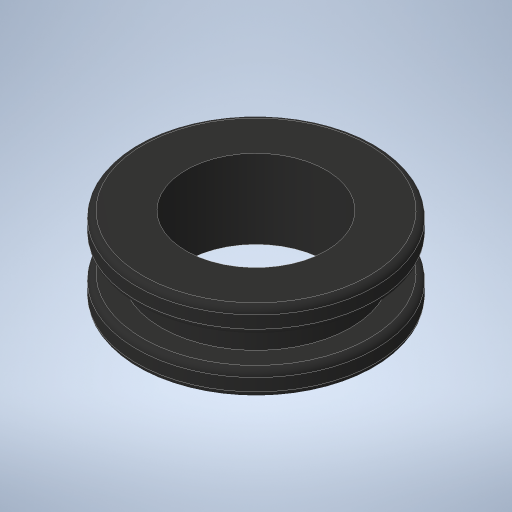
# Autodesk Inventor part: .5 tpu grommet
Saved by Autodesk Inventor 2023.4 (Build 274418000, 418)
## iProperties
Created: 2025-03-24
Part Number: .5 tpu grommet
Material: Rubber, Black
Document SubType Name: Modeling
Designer: jmcintyr
Density: 0.93 g/cm^3
Appearance: Rubber - Black
Author: jmcintyr
Autodesk Inventor part; units mm, degrees
ref_plane "YZ Plane" through (0, 0, 0) normal (1, 0, 0) x (0, 1, 0)
ref_plane "XZ Plane" through (0, 0, 0) normal (0, 1, 0) x (-1, 0, 0)
ref_plane "XY Plane" through (0, 0, 0) normal (0, 0, 1) x (1, 0, 0)
sketch "Sketch1" plane through (0, 0, 0) normal (0, 0, 1) x (1, 0, 0)
  line L0 (4.5085, 2.54) -> (4.5085, -2.54)
  line L1 (4.5085, -2.54) -> (7.6835, -2.54)
  line L2 (7.6835, -2.54) -> (7.6835, -0.9525)
  line L3 (7.6835, -0.9525) -> (6.096, -0.9525)
  line L4 (6.096, -0.9525) -> (6.096, 0.9525)
  line L5 (6.096, 0.9525) -> (7.6835, 0.9525)
  line L6 (7.6835, 0.9525) -> (7.6835, 2.54)
  line L7 (7.6835, 2.54) -> (4.5085, 2.54)
  line L8 (0, 0) -> (0, 2.54) construction
  point P0 (4.5085, 0)
  point P1 (6.096, 0)
  dimension "d0" = 6.096
  dimension "d1" = 1.905
  dimension "d2" = 5.08
  dimension "d3" = 1.5875
  dimension "d4" = 1.5875
  dimension "d5" = 1.5875
  constraints: 18 end point, 7 perpendicular, 3 horizontal alignment, 2 midpoint, 2 vertical, 1 vertical alignment
  measures "d0" distance from line of L8.start L4
  measures "d1" distance of L3.end L4.end
  measures "d2" distance of L0.start L0.end
  measures "d3" distance of L5.end L6.end
  measures "d4" distance between parallel lines of L4 L0
  measures "d5" distance of L2.end L3.end
revolve "Revolution1" add sketch "Sketch1" angle 360 about axis through (0, 0, 0) along (0, 1, 0)
fillet "Fillet1" radius 0.3969 4 edges at (-7.6835, -0.9525, 0) (-7.6835, -2.54, 0) (-7.6835, 0.9525, 0) (-7.6835, 2.54, 0)
equation "\"d4\" = d3"
body "Solid1"
